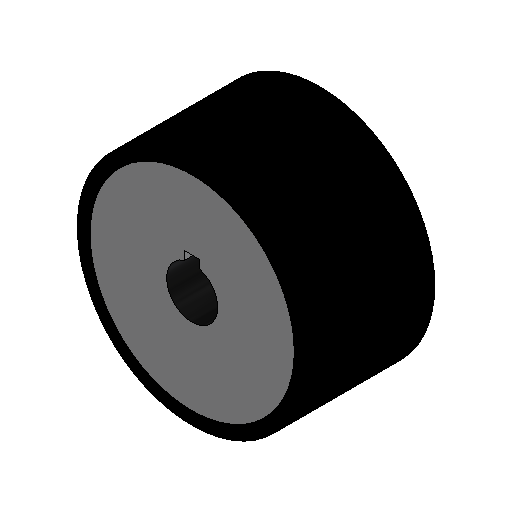
# Autodesk Inventor part: TL20240701-10110CV-009
Saved by Autodesk Inventor 2022.5 (Build 265521000, 521)
## iProperties
Category: DRIVE UNIT ASSY
Company: 현대 트랜시스(대유)
Created: 2023-02-03
Part Number: TL20240701-10110CV-009
Project: SW PJT
Checked By: 김형민
Engr Approved By: 김시현
Material: S45C
Description: 0
Document SubType Name: Modeling
Mfg Approved By: 호상태
Designer: 박성규
Mass: 1262.03 g
Surface Area: 814.222 cm^2
Volume: 467.417 cm^3
Density: 7.87 g/cm^3
Appearance: Anodizing White
Stock Number: 009
User Status: 2 x18
DETAIL: Coveryor Assembly
M/C TITLE: MEa/NEa차종 시트조립라인
PARTS NAME: Bracket
SPECIFICATION: TA20221101-CV200000-015
DocNumber: 221118_Standard_v1
Folder: .\
VDS_Category: 엔지니어링
Detail Description: Processed products
Title: IDLE ROLLER
Subject: SW차종 시트조립라인
Author: 박성규
Revision Number: A
Autodesk Inventor part; units mm, degrees
ref_plane "YZ Plane" through (0, 0, 0) normal (1, 0, 0) x (0, 1, 0)
ref_plane "XZ Plane" through (0, 0, 0) normal (0, 1, 0) x (-1, 0, 0)
ref_plane "XY Plane" through (0, 0, 0) normal (0, 0, 1) x (1, 0, 0)
sketch "스케치9" plane through (0, 0, 0) normal (0, 0, 1) x (1, 0, 0)
  circle A0 centre (0, 0) radius 40
  dimension "d40" = 80
  constraints: 1 centre point, 1 coincident
  measures "d40" diameter of A0
extrude "돌출4" add sketch "스케치9" along normal mid plane 50
sketch "스케치10" plane through (0, 0, 25) normal (0, 0, 1) x (1, 0, 0)
  circle A0 centre (0, 0) radius 40 construction
  constraints: 1 coincident
hole "구멍3" at (0, 0, 25) direction (0, 0, -1) diameter 20 end through all
sketch "스케치11" plane through (0, 0, 25) normal (0, 0, 1) x (1, 0, 0)
  circle A0 centre (0, 0) radius 10 construction
  line L0 (-3, 12.8) -> (3, 12.8)
  line L1 (3, 12.8) -> (3, 6.8)
  line L2 (3, 6.8) -> (-3, 6.8)
  line L3 (-3, 6.8) -> (-3, 12.8)
  line L4 (-3, 12.8) -> (3, 6.8) construction
  line L5 (3, 12.8) -> (-3, 6.8) construction
  point P0 (0, 9.8)
  point P1 (0, 9.8)
  dimension "d50" = 12.8
  dimension "d51" = 6
  dimension "d52" = 6
  constraints: 12 end point, 3 midpoint, 2 parallel, 1 horizontal, 1 perpendicular, 1 vertical alignment
  measures "d50" distance from line of A0.centre L0
  measures "d51" distance of L0.end L1.end
  measures "d52" distance of L0.start L0.end
extrude "돌출5" cut sketch "스케치11" against normal blind 80
sketch "스케치12" plane through (0, 0, 0) normal (0, 0, 1) x (1, 0, 0)
  circle A0 centre (0, 0) radius 45
  circle A1 centre (0, 0) radius 40 projected
  dimension "d55" = 90
  constraints: 1 centre point, 1 coincident
  measures "d55" diameter of A0
extrude "돌출6" add sketch "스케치12" along normal mid plane 50 separate body
